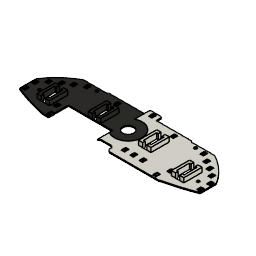
Amaturenbrett_Auto (Autodesk Fusion 360 design; units mm, degrees)
Autodesk Fusion 360 part; units mm, degrees
sketch "Skizze1" plane through (0, 0, 0) normal (0, 0, 1) x (1, 0, 0)
  line L0 (0, 10) -> (-10, 10)
  line L1 (-10, 10) -> (-13, 7)
  line L2 (-13, 7) -> (-13, 2)
  line L3 (-13, 2) -> (-15, 0)
  spline S0 degree 5 poles (-110, 0) (-110.1613, 0.0605) (-110.7348, 0.2373) (-112.3477, 0.67) (-115.9134, 1.5732) (-122.2237, 3.1932) (-129.7281, 5.2238) (-137.7121, 7.5525) (-145.4822, 10.0264) (-152.4484, 12.4304) (-158.1215, 14.5178) (-161.3098, 15.7444) (-162.8158, 16.3309) (-163.4105, 16.5624) (-163.6056, 16.6383) knots 0 0 0 0 0 0 0.1 0.2 0.3 0.4 0.5 0.6 0.7 0.8 0.9 1 1 1 1 1 1
  line L4 (-163.6056, 16.6383) -> (-163.6056, 46)
  spline S1 degree 5 poles (-163.6056, 46) (-163.4847, 46.1973) (-163.1089, 46.8) (-162.1433, 48.3283) (-160.053, 51.5223) (-156.1277, 56.9302) (-150.9771, 63.1091) (-144.7998, 69.3982) (-137.996, 75.2415) (-131.2216, 80.2701) (-125.2328, 84.2311) (-121.6617, 86.4119) (-119.9315, 87.445) (-119.2344, 87.8605) (-119, 88) knots 0 0 0 0 0 0 0.1 0.2 0.3 0.4 0.5 0.6 0.7 0.8 0.9 1 1 1 1 1 1
  line L5 (-119, 88) -> (-77, 88)
  line L6 (-77, 88) -> (-75, 90)
  line L7 (-75, 90) -> (-11, 90)
  line L8 (-11, 90) -> (-11, 99)
  line L9 (-11, 99) -> (-9.3607, 100.6393)
  line L10 (-9.3607, 100.6393) -> (0, 100.6393)
  line L11 (0, 1.75) -> (0, 22.5)
  line L12 (13, 2) -> (16.5, -1.5)
  line L13 (75, 90) -> (11, 90)
  line L14 (119, 88) -> (77, 88)
  spline S2 degree 5 poles (104.5, -1.5) (104.7668, -1.4344) (105.5646, -1.2376) (107.5534, -0.7459) (111.692, 0.289) (118.7937, 2.1326) (127.1068, 4.4102) (135.8553, 6.9754) (144.2868, 9.6506) (151.7717, 12.2139) (157.8159, 14.417) (161.1893, 15.7031) (162.777, 16.3168) (163.4017, 16.559) (163.6056, 16.6383) knots 0 0 0 0 0 0 0.1 0.2 0.3 0.4 0.5 0.6 0.7 0.8 0.9 1 1 1 1 1 1
  line L15 (-106, -1.5) -> (-114, 1.5)
  line L16 (-158.3876, 14.6077) -> (-168.8236, 18.669)
  line L17 (98.7017, -2.9261) -> (110.2983, -0.0739)
  line L18 (158.3876, 14.6077) -> (168.8236, 18.669)
  spline S3 degree 5 poles (163.6056, 46) (163.4847, 46.1973) (163.1089, 46.8) (162.1433, 48.3283) (160.053, 51.5223) (156.1277, 56.9302) (150.9771, 63.1091) (144.7998, 69.3982) (137.996, 75.2415) (131.2216, 80.2701) (125.2328, 84.2311) (121.6617, 86.4119) (119.9315, 87.445) (119.2344, 87.8605) (119, 88) knots 0 0 0 0 0 0 0.1 0.2 0.3 0.4 0.5 0.6 0.7 0.8 0.9 1 1 1 1 1 1
  line L19 (-167.0116, 40.4408) -> (-160.1996, 51.5592)
  line L20 (-125.039, 84.4076) -> (-112.961, 91.5924)
  line L21 (167.0116, 40.4408) -> (160.1996, 51.5592)
  line L22 (125.039, 84.4076) -> (112.961, 91.5924)
  line L23 (77, 88) -> (75, 90)
  line L24 (10, 10) -> (13, 7)
  line L25 (163.6056, 16.6383) -> (163.6056, 46)
  line L26 (16.5, -1.5) -> (104.5, -1.5)
  line L27 (11, 99) -> (9.3607, 100.6393)
  line L28 (13, 7) -> (13, 2)
  line L29 (0, 10) -> (10, 10)
  line L30 (9.3607, 100.6393) -> (0, 100.6393)
  line L31 (11, 90) -> (11, 99)
  circle A0 centre (-158.8575, 41.2647) radius 1.75
  circle A1 centre (-158.8575, 23.2647) radius 1.75
  circle A2 centre (-147.7393, 54.3878) radius 1.75
  circle A3 centre (-120.4151, 72.4981) radius 1.75
  circle A4 centre (158.8575, 23.2647) radius 1.75
  circle A5 centre (158.8575, 41.2647) radius 1.75
  circle A6 centre (0, 50) radius 25
  line L32 (11, 90) -> (11, 72.4499)
  line L33 (13, 7) -> (13, 28.6458)
  circle A7 centre (0, 50) radius 10
  circle A8 centre (-89.5, 82.5) radius 2.75
  circle A9 centre (143.3281, 32.327) radius 2.5
  circle A10 centre (-144.409, 32.4498) radius 2.5
  line L34 (-146.8803, 32.0722) -> (-144.8803, 32.0722)
  line L35 (-142.4192, 30.1189) -> (-142.2776, 30.1189)
  circle A11 centre (-106, 82) radius 1.75
  circle A12 centre (-103, 25) radius 1.75
  circle A13 centre (-95.8089, 4.2466) radius 1.75
  circle A14 centre (-45, 46) radius 5
  circle A15 centre (120.3035, 27.3959) radius 5
  line L36 (21.162, 34.5574) -> (76.9201, 34.5574)
  line L37 (76.9201, 34.5574) -> (76.9201, 2.4702)
  line L38 (76.9201, 2.4702) -> (21.162, 2.4702)
  line L39 (21.162, 2.4702) -> (21.162, 34.5574)
  line L40 (-110, 0) -> (-106, -1.5)
  line L41 (-106, -1.5) -> (-17, -1.5)
  line L42 (-17, -1.5) -> (-15, 0)
  circle A16 centre (-134.5283, 64.1132) radius 1.75
  line L43 (-161.8015, 26.3684) -> (-155.8015, 26.3684)
  line L44 (-155.8015, 26.3684) -> (-155.8015, 20.3684)
  line L45 (-155.8015, 20.3684) -> (-161.8015, 20.3684)
  line L46 (-161.8015, 20.3684) -> (-161.8015, 26.3684)
  line L47 (-161.7377, 38.3687) -> (-161.7377, 44.3687)
  line L48 (-161.7377, 44.3687) -> (-155.7377, 44.3687)
  line L49 (-155.7377, 44.3687) -> (-155.7377, 38.3687)
  line L50 (-155.7377, 38.3687) -> (-161.7377, 38.3687)
  line L51 (-131.5751, 61.1788) -> (-137.5751, 61.1788)
  line L52 (-137.5751, 61.1788) -> (-137.5751, 67.1788)
  line L53 (-137.5751, 67.1788) -> (-131.5751, 67.1788)
  line L54 (-131.5751, 67.1788) -> (-131.5751, 61.1788)
  line L55 (-123.3948, 69.6725) -> (-123.3948, 75.6725)
  line L56 (-123.3948, 75.6725) -> (-117.3948, 75.6725)
  line L57 (-117.3948, 75.6725) -> (-117.3948, 69.6725)
  line L58 (-117.3948, 69.6725) -> (-123.3948, 69.6725)
  line L59 (-108.9492, 79.0086) -> (-108.9492, 85.0086)
  line L60 (-108.9492, 85.0086) -> (-102.9492, 85.0086)
  line L61 (-102.9492, 85.0086) -> (-102.9492, 79.0086)
  line L62 (-102.9492, 79.0086) -> (-108.9492, 79.0086)
  line L63 (-106.0964, 22.0509) -> (-106.0964, 28.0509)
  line L64 (-106.0964, 28.0509) -> (-100.0964, 28.0509)
  line L65 (-100.0964, 28.0509) -> (-100.0964, 22.0509)
  line L66 (-100.0964, 22.0509) -> (-106.0964, 22.0509)
  line L67 (-98.7463, 7.3835) -> (-92.7463, 7.3835)
  line L68 (-92.7463, 7.3835) -> (-92.7463, 1.3835)
  line L69 (-92.7463, 1.3835) -> (-98.7463, 1.3835)
  line L70 (-98.7463, 1.3835) -> (-98.7463, 7.3835)
  circle A17 centre (-61.0017, 16.9954) radius 1.75
  line L71 (-63.9392, 13.9164) -> (-63.9392, 19.9164)
  line L72 (-57.9392, 13.9164) -> (-63.9392, 13.9164)
  line L73 (-57.9392, 19.9164) -> (-57.9392, 13.9164)
  line L74 (-63.9392, 19.9164) -> (-57.9392, 19.9164)
  circle A18 centre (-44.4166, 16.9103) radius 1.75
  circle A19 centre (-28.1708, 16.8342) radius 1.75
  line L75 (3.0172, 92.0677) -> (-2.9828, 92.0677)
  line L76 (-2.9828, 92.0677) -> (-2.9828, 98.0677)
  line L77 (-2.9828, 98.0677) -> (3.0172, 98.0677)
  line L78 (3.0172, 98.0677) -> (3.0172, 92.0677)
  circle A20 centre (0.0266, 95.0028) radius 1.75
  line L79 (-48.3744, 79.3302) -> (-54.3744, 79.3302)
  line L80 (-54.3744, 79.3302) -> (-54.3744, 85.3302)
  line L81 (-54.3744, 85.3302) -> (-48.3744, 85.3302)
  line L82 (-48.3744, 85.3302) -> (-48.3744, 79.3302)
  circle A21 centre (-51.3653, 82.3011) radius 1.75
  line L83 (47.6167, 79.2941) -> (47.6167, 85.2941)
  line L84 (47.6167, 85.2941) -> (53.6167, 85.2941)
  line L85 (53.6167, 85.2941) -> (53.6167, 79.2941)
  line L86 (53.6167, 79.2941) -> (47.6167, 79.2941)
  circle A22 centre (50.6982, 82.3011) radius 1.75
  circle A23 centre (89.1589, 82.4646) radius 2.5
  line L87 (102.0349, 78.6834) -> (102.0349, 84.6834)
  line L88 (102.0349, 84.6834) -> (108.0349, 84.6834)
  line L89 (108.0349, 84.6834) -> (108.0349, 78.6834)
  line L90 (108.0349, 78.6834) -> (102.0349, 78.6834)
  circle A24 centre (105.0444, 81.6905) radius 1.75
  line L91 (117.3503, 69.6133) -> (117.3503, 75.6133)
  line L92 (117.3503, 75.6133) -> (123.3503, 75.6133)
  line L93 (123.3503, 75.6133) -> (123.3503, 69.6133)
  line L94 (123.3503, 69.6133) -> (117.3503, 69.6133)
  circle A25 centre (120.4318, 72.5126) radius 1.75
  line L95 (130.8921, 61.2538) -> (130.8921, 67.2538)
  line L96 (130.8921, 67.2538) -> (136.8921, 67.2538)
  line L97 (136.8921, 67.2538) -> (136.8921, 61.2538)
  line L98 (136.8921, 61.2538) -> (130.8921, 61.2538)
  circle A26 centre (133.8942, 64.189) radius 1.75
  line L99 (150.7504, 51.4949) -> (144.7504, 51.4949)
  line L100 (144.7504, 51.4949) -> (144.7504, 57.4949)
  line L101 (144.7504, 57.4949) -> (150.7504, 57.4949)
  line L102 (150.7504, 57.4949) -> (150.7504, 51.4949)
  circle A27 centre (147.7239, 54.3795) radius 1.75
  line L103 (161.805, 38.5537) -> (155.805, 38.5537)
  line L104 (155.805, 38.5537) -> (155.805, 44.5537)
  line L105 (155.805, 44.5537) -> (161.805, 44.5537)
  line L106 (161.805, 44.5537) -> (161.805, 38.5537)
  line L107 (155.874, 26.4991) -> (161.874, 26.4991)
  line L108 (161.874, 26.4991) -> (161.874, 20.4991)
  line L109 (155.874, 20.4991) -> (155.874, 26.4991)
  line L110 (161.874, 20.4991) -> (155.874, 20.4991)
  circle A28 centre (95.7662, 4.2772) radius 1.75
  line L111 (92.7927, 7.3926) -> (98.7927, 7.3926)
  line L112 (98.7927, 7.3926) -> (98.7927, 1.3926)
  line L113 (92.7927, 1.3926) -> (92.7927, 7.3926)
  line L114 (98.7927, 1.3926) -> (92.7927, 1.3926)
  line L115 (106.0344, 22.2433) -> (100.0344, 22.2433)
  line L116 (100.0344, 22.2433) -> (100.0344, 28.2433)
  line L117 (100.0344, 28.2433) -> (106.0344, 28.2433)
  line L118 (106.0344, 28.2433) -> (106.0344, 22.2433)
  circle A29 centre (103.0079, 25.128) radius 1.75
  line L119 (-144.7191, 51.5389) -> (-150.7191, 51.5389)
  line L120 (-150.7191, 51.5389) -> (-150.7191, 57.5389)
  line L121 (-150.7191, 57.5389) -> (-144.7191, 57.5389)
  line L122 (-144.7191, 57.5389) -> (-144.7191, 51.5389)
  line L123 (-41.4351, 13.9164) -> (-47.4351, 13.9164)
  line L124 (-47.4351, 13.9164) -> (-47.4351, 19.9164)
  line L125 (-47.4351, 19.9164) -> (-41.4351, 19.9164)
  line L126 (-41.4351, 19.9164) -> (-41.4351, 13.9164)
  line L127 (-25.4351, 13.9164) -> (-31.4351, 13.9164)
  line L128 (-31.4351, 13.9164) -> (-31.4351, 19.9164)
  line L129 (-31.4351, 19.9164) -> (-25.4351, 19.9164)
  line L130 (-25.4351, 19.9164) -> (-25.4351, 13.9164)
  line L131 (-38.3249, 39.7163) -> (-51.8249, 39.7163)
  line L132 (-51.8249, 39.7163) -> (-51.8249, 63.2163)
  line L133 (-51.8249, 63.2163) -> (-38.3249, 63.2163)
  line L134 (-38.3249, 63.2163) -> (-38.3249, 39.7163)
  line L135 (-38.3249, 39.9465) -> (-38.3249, 63.2163)
  line L136 (-56.2684, 39.9376) -> (-56.2684, 62.9381)
  line L137 (-33.7684, 67.9381) -> (-56.2684, 67.9381)
  line L138 (-56.2684, 67.9381) -> (-56.2684, 62.9381)
  line L139 (-33.7684, 34.9376) -> (-56.2684, 34.9376)
  line L140 (-56.2684, 34.9376) -> (-56.2684, 39.9376)
  line L141 (-33.7684, 67.9381) -> (-56.2684, 67.9381)
  line L142 (-56.2684, 67.9381) -> (-56.2684, 62.9381)
  line L143 (-56.2684, 34.9376) -> (-56.2684, 39.9376)
  line L144 (-33.7684, 34.9376) -> (-56.2684, 34.9376)
  line L145 (-33.7684, 34.9376) -> (-33.7684, 67.9381)
  line L146 (39.1751, 39.7163) -> (39.1751, 63.2163)
  line L147 (39.1751, 63.2163) -> (52.6751, 63.2163)
  line L148 (34.7316, 34.9376) -> (34.7316, 39.9376)
  line L149 (57.2316, 34.9376) -> (34.7316, 34.9376)
  line L150 (52.6751, 63.2163) -> (52.6751, 39.7163)
  line L151 (57.2316, 67.9381) -> (34.7316, 67.9381)
  line L152 (57.2316, 34.9376) -> (57.2316, 67.9381)
  line L153 (52.6751, 39.7163) -> (39.1751, 39.7163)
  circle A30 centre (46, 46) radius 5
  line L154 (34.7316, 39.9376) -> (34.7316, 62.9381)
  line L155 (34.7316, 67.9381) -> (34.7316, 62.9381)
  line L156 (57.2316, 67.9381) -> (34.7316, 67.9381)
  line L157 (57.2316, 34.9376) -> (34.7316, 34.9376)
  line L158 (34.7316, 34.9376) -> (34.7316, 39.9376)
  line L159 (52.6751, 39.9465) -> (52.6751, 63.2163)
  line L160 (34.7316, 67.9381) -> (34.7316, 62.9381)
  line L161 (-33.7684, 34.9376) -> (-33.7684, 67.9381)
  line L162 (-33.7684, 34.9376) -> (-56.2684, 34.9376)
  line L163 (-56.2684, 34.9376) -> (-56.2684, 39.9376)
  line L164 (-56.2684, 39.9376) -> (-56.2684, 62.9381)
  line L165 (-56.2684, 67.9381) -> (-56.2684, 62.9381)
  line L166 (-33.7684, 67.9381) -> (-56.2684, 67.9381)
  line L167 (-38.3249, 63.2163) -> (-38.3249, 39.7163)
  line L168 (-51.8249, 39.7163) -> (-51.8249, 63.2163)
  line L169 (-51.8249, 63.2163) -> (-38.3249, 63.2163)
  line L170 (-38.3249, 39.7163) -> (-51.8249, 39.7163)
  line L171 (-33.7684, 34.9376) -> (-33.7684, 67.9381)
  line L172 (-33.7684, 34.9376) -> (-56.2684, 34.9376)
  line L173 (-56.2684, 34.9376) -> (-56.2684, 39.9376)
  line L174 (-56.2684, 39.9376) -> (-56.2684, 62.9381)
  line L175 (-56.2684, 67.9381) -> (-56.2684, 62.9381)
  line L176 (-33.7684, 67.9381) -> (-56.2684, 67.9381)
  line L177 (-51.8249, 63.2163) -> (-38.3249, 63.2163)
  line L178 (-38.3249, 63.2163) -> (-38.3249, 39.7163)
  line L179 (-51.8249, 39.7163) -> (-51.8249, 63.2163)
  line L180 (-38.3249, 39.7163) -> (-51.8249, 39.7163)
  circle A31 centre (-122.3546, 28.1544) radius 5
  line L181 (-133.6684, 17.0376) -> (-133.6684, 22.0376)
  line L182 (-133.6684, 20.0376) -> (-133.6684, 45.0381)
  line L183 (-133.6684, 50.0381) -> (-133.6684, 45.0381)
  line L184 (-111.1684, 50.0381) -> (-133.6684, 50.0381)
  line L185 (-111.1684, 17.0376) -> (-111.1684, 50.0381)
  line L186 (-111.1684, 17.0376) -> (-133.6684, 17.0376)
  line L187 (-133.6684, 15.0376) -> (-133.6684, 20.0376)
  line L188 (-129.2249, 45.3163) -> (-115.7249, 45.3163)
  line L189 (-115.7249, 45.3163) -> (-115.7249, 21.8163)
  line L190 (-129.2249, 21.8163) -> (-129.2249, 45.3163)
  line L191 (-115.7249, 21.8163) -> (-129.2249, 21.8163)
  line L192 (109.0526, 21.3481) -> (109.0526, 44.3486)
  line L193 (109.0526, 16.3481) -> (109.0526, 21.3481)
  line L194 (131.5526, 16.3481) -> (109.0526, 16.3481)
  line L195 (131.5526, 16.3481) -> (131.5526, 49.3486)
  line L196 (131.5526, 49.3486) -> (109.0526, 49.3486)
  line L197 (109.0526, 49.3486) -> (109.0526, 44.3486)
  line L198 (126.9961, 21.1268) -> (113.4961, 21.1268)
  line L199 (113.4961, 21.1268) -> (113.4961, 44.6268)
  line L200 (113.4961, 44.6268) -> (126.9961, 44.6268)
  line L201 (126.9961, 44.6268) -> (126.9961, 21.1268)
  line L202 (116.5254, 44.6268) -> (116.5254, 49.3486)
  line L203 (123.9565, 44.6268) -> (123.9565, 49.3486)
  line L204 (116.5254, 44.6268) -> (116.5254, 16.3481)
  line L205 (123.9565, 49.3486) -> (123.9565, 16.3481)
  line L206 (120.2461, 44.6268) -> (116.5461, 44.6268)
  line L207 (123.9565, 44.6268) -> (123.9565, 49.3486)
  line L208 (123.9565, 49.3486) -> (123.9565, 16.3481)
  line L209 (116.5254, 44.6268) -> (116.5254, 49.3486)
  line L210 (116.5254, 44.6268) -> (116.5254, 16.3481)
  line L211 (45.9251, 63.2163) -> (49.6251, 63.2163)
  line L212 (45.9251, 63.2163) -> (42.2251, 63.2163)
  line L213 (42.2251, 63.2163) -> (42.2251, 67.9381)
  line L214 (42.2251, 67.9381) -> (42.2251, 34.9376)
  line L215 (49.6251, 67.9381) -> (49.6251, 34.9376)
  line L216 (-45.0184, 67.9381) -> (-48.7184, 67.9381)
  line L217 (-45.0184, 67.9381) -> (-41.3184, 67.9381)
  line L218 (-41.3184, 67.9381) -> (-41.3184, 34.9376)
  line L219 (-48.7184, 67.9381) -> (-48.7184, 34.9376)
  line L220 (-122.4184, 50.0381) -> (-126.1184, 50.0381)
  line L221 (-122.4184, 50.0381) -> (-118.7184, 50.0381)
  line L222 (-126.1184, 50.0381) -> (-126.1184, 17.0376)
  line L223 (-118.7184, 50.0381) -> (-118.7184, 17.0376)
  line L224 (13, -1.5) -> (92.9118, -1.5)
  line L225 (92.9118, -1.5) -> (92.9118, 34.5574)
  line L226 (92.9118, 34.5574) -> (13, 34.5574)
  line L227 (13, 34.5574) -> (13, -1.5)
  line L228 (-54.3744, 79.3302) -> (-48.3744, 79.3302)
  line L229 (-48.3744, 79.3302) -> (-48.3744, 77.3302)
  line L230 (-48.3744, 77.3302) -> (-54.3744, 77.3302)
  line L231 (-54.3744, 77.3302) -> (-54.3744, 79.3302)
  line L232 (-102.9492, 79.0086) -> (-108.9492, 79.0086)
  line L233 (-108.9492, 79.0086) -> (-108.9492, 77.0086)
  line L234 (-108.9492, 77.0086) -> (-102.9492, 77.0086)
  line L235 (-102.9492, 77.0086) -> (-102.9492, 79.0086)
  line L236 (-117.3948, 69.6725) -> (-123.3948, 69.6725)
  line L237 (-123.3948, 69.6725) -> (-123.3948, 67.6725)
  line L238 (-123.3948, 67.6725) -> (-117.3948, 67.6725)
  line L239 (-117.3948, 67.6725) -> (-117.3948, 69.6725)
  line L240 (-131.5751, 61.1788) -> (-137.5751, 61.1788)
  line L241 (-137.5751, 61.1788) -> (-137.5751, 59.1788)
  line L242 (-137.5751, 59.1788) -> (-131.5751, 59.1788)
  line L243 (-131.5751, 59.1788) -> (-131.5751, 61.1788)
  line L244 (-144.7191, 51.5389) -> (-150.7191, 51.5389)
  line L245 (-150.7191, 51.5389) -> (-150.7191, 49.5389)
  line L246 (-150.7191, 49.5389) -> (-144.7191, 49.5389)
  line L247 (-144.7191, 49.5389) -> (-144.7191, 51.5389)
  line L248 (-155.7377, 38.3687) -> (-161.7377, 38.3687)
  line L249 (-161.7377, 38.3687) -> (-161.7377, 36.3687)
  line L250 (-161.7377, 36.3687) -> (-155.7377, 36.3687)
  line L251 (-155.7377, 36.3687) -> (-155.7377, 38.3687)
  line L252 (-155.8015, 20.3684) -> (-161.8015, 20.3684)
  line L253 (-161.8015, 20.3684) -> (-161.8015, 18.3684)
  line L254 (-161.8015, 18.3684) -> (-155.8015, 18.3684)
  line L255 (-155.8015, 18.3684) -> (-155.8015, 20.3684)
  line L256 (-100.0964, 22.0509) -> (-106.0964, 22.0509)
  line L257 (-106.0964, 22.0509) -> (-106.0964, 20.0509)
  line L258 (-106.0964, 20.0509) -> (-100.0964, 20.0509)
  line L259 (-100.0964, 20.0509) -> (-100.0964, 22.0509)
  line L260 (-92.7463, 7.3835) -> (-98.7463, 7.3835)
  line L261 (-98.7463, 7.3835) -> (-98.7463, 9.3835)
  line L262 (-98.7463, 9.3835) -> (-92.7463, 9.3835)
  line L263 (-92.7463, 9.3835) -> (-92.7463, 7.3835)
  line L264 (-63.9392, 13.9164) -> (-57.9392, 13.9164)
  line L265 (-57.9392, 13.9164) -> (-57.9392, 11.9164)
  line L266 (-57.9392, 11.9164) -> (-63.9392, 11.9164)
  line L267 (-63.9392, 11.9164) -> (-63.9392, 13.9164)
  line L268 (-47.4351, 13.9164) -> (-41.4351, 13.9164)
  line L269 (-41.4351, 13.9164) -> (-41.4351, 11.9164)
  line L270 (-41.4351, 11.9164) -> (-47.4351, 11.9164)
  line L271 (-47.4351, 11.9164) -> (-47.4351, 13.9164)
  line L272 (-31.4351, 13.9164) -> (-25.4351, 13.9164)
  line L273 (-25.4351, 13.9164) -> (-25.4351, 11.9164)
  line L274 (-25.4351, 11.9164) -> (-31.4351, 11.9164)
  line L275 (-31.4351, 11.9164) -> (-31.4351, 13.9164)
  line L276 (47.6167, 79.2941) -> (53.6167, 79.2941)
  line L277 (53.6167, 79.2941) -> (53.6167, 77.2941)
  line L278 (53.6167, 77.2941) -> (47.6167, 77.2941)
  line L279 (47.6167, 77.2941) -> (47.6167, 79.2941)
  line L280 (102.0349, 78.6834) -> (108.0349, 78.6834)
  line L281 (108.0349, 78.6834) -> (108.0349, 76.6834)
  line L282 (108.0349, 76.6834) -> (102.0349, 76.6834)
  line L283 (102.0349, 76.6834) -> (102.0349, 78.6834)
  line L284 (117.3503, 69.6133) -> (123.3503, 69.6133)
  line L285 (123.3503, 69.6133) -> (123.3503, 67.6133)
  line L286 (123.3503, 67.6133) -> (117.3503, 67.6133)
  line L287 (117.3503, 67.6133) -> (117.3503, 69.6133)
  line L288 (130.8921, 61.2538) -> (136.8921, 61.2538)
  line L289 (136.8921, 61.2538) -> (136.8921, 59.2538)
  line L290 (136.8921, 59.2538) -> (130.8921, 59.2538)
  line L291 (130.8921, 59.2538) -> (130.8921, 61.2538)
  line L292 (144.7504, 51.4949) -> (150.7504, 51.4949)
  line L293 (150.7504, 51.4949) -> (150.7504, 49.4949)
  line L294 (150.7504, 49.4949) -> (144.7504, 49.4949)
  line L295 (144.7504, 49.4949) -> (144.7504, 51.4949)
  line L296 (155.805, 38.5537) -> (161.805, 38.5537)
  line L297 (161.805, 38.5537) -> (161.805, 36.5537)
  line L298 (161.805, 36.5537) -> (155.805, 36.5537)
  line L299 (155.805, 36.5537) -> (155.805, 38.5537)
  line L300 (155.874, 20.4991) -> (161.874, 20.4991)
  line L301 (161.874, 20.4991) -> (161.874, 18.4991)
  line L302 (161.874, 18.4991) -> (155.874, 18.4991)
  line L303 (155.874, 18.4991) -> (155.874, 20.4991)
  line L304 (100.0344, 22.2433) -> (106.0344, 22.2433)
  line L305 (106.0344, 22.2433) -> (106.0344, 20.2433)
  line L306 (106.0344, 20.2433) -> (100.0344, 20.2433)
  line L307 (100.0344, 20.2433) -> (100.0344, 22.2433)
  line L308 (98.7927, 7.3926) -> (92.7927, 7.3926)
  line L309 (92.7927, 7.3926) -> (92.7927, 9.3926)
  line L310 (92.7927, 9.3926) -> (98.7927, 9.3926)
  line L311 (98.7927, 9.3926) -> (98.7927, 7.3926)
  line L312 (3.0172, 92.0677) -> (-2.9828, 92.0677)
  line L313 (-2.9828, 92.0677) -> (-2.9828, 90.0677)
  line L314 (-2.9828, 90.0677) -> (3.0172, 90.0677)
  line L315 (3.0172, 90.0677) -> (3.0172, 92.0677)
  point P0 (-139, 8)
  point P1 (-146, 68)
  point P2 (146, 68)
  point P3 (139, 8)
  point P4 (-120.6376, 72.9849)
  point P5 (-85, 76)
  point P6 (-120.6376, 72.9849)
  dimension "d3" = 3.5
  dimension "d4" = 3.5
  dimension "d5" = 3.5
  dimension "d6" = 3.5
  dimension "d15" = 20
  dimension "d23" = 5.5
  dimension "d35" = 5
  dimension "d37" = 2
  dimension "d38" = 5
  dimension "d39" = 3.5
  dimension "d41" = 3.5
  dimension "d46" = 3.5
  dimension "d52" = 10
  dimension "d54" = 10
  dimension "d55" = 3.5
  dimension "d60" = 6
  dimension "d61" = 6
  dimension "d62" = 6
  dimension "d63" = 6
  dimension "d66" = 6
  dimension "d67" = 6
  dimension "d68" = 6
  dimension "d69" = 6
  dimension "d70" = 6
  dimension "d71" = 6
  dimension "d72" = 6
  dimension "d73" = 6
  dimension "d74" = 6
  dimension "d75" = 6
  dimension "d76" = 3.5
  dimension "d77" = 6
  dimension "d78" = 6
  dimension "d79" = 3.5
  dimension "d82" = 3.5
  dimension "d85" = 3.5
  dimension "d86" = 6
  dimension "d87" = 6
  dimension "d88" = 3.5
  dimension "d89" = 6
  dimension "d90" = 6
  dimension "d91" = 3.5
  dimension "d92" = 6
  dimension "d93" = 6
  dimension "d94" = 5
  dimension "d97" = 3.5
  dimension "d98" = 6
  dimension "d99" = 6
  dimension "d100" = 3.5
  dimension "d101" = 6
  dimension "d102" = 6
  dimension "d103" = 3.5
  dimension "d104" = 6
  dimension "d105" = 6
  dimension "d106" = 3.5
  dimension "d107" = 6
  dimension "d108" = 6
  dimension "d109" = 6
  dimension "d110" = 6
  dimension "d111" = 6
  dimension "d112" = 6
  dimension "d113" = 3.5
  dimension "d114" = 6
  dimension "d115" = 6
  dimension "d116" = 3.5
  dimension "d117" = 6
  dimension "d118" = 6
  dimension "d137" = 6
  dimension "d138" = 6
  dimension "d139" = 6
  dimension "d140" = 6
  dimension "d141" = 6
  dimension "d142" = 6
  dimension "d149" = 13.5
  dimension "d150" = 23.5
  dimension "d160" = 5
  dimension "d162" = 5
  dimension "d164" = 5
  dimension "d166" = 5
  dimension "d171" = 10
  dimension "d172" = 13.5
  dimension "d173" = 23.5
  dimension "d174" = 5
  dimension "d175" = 5
  dimension "d176" = 5
  dimension "d177" = 5
  dimension "d180" = 13.5
  dimension "d181" = 23.5
  dimension "d182" = 5
  dimension "d183" = 5
  dimension "d184" = 10
  dimension "d185" = 13.5
  dimension "d186" = 23.5
  dimension "d187" = 5
  dimension "d188" = 5
  dimension "d190" = 5
  dimension "d191" = 5
  dimension "d192" = 5
  dimension "d193" = 13.5
  dimension "d194" = 23.5
  dimension "d196" = 13.5
  dimension "d197" = 23.5
  dimension "d198" = 5
  dimension "d199" = 5
  dimension "d200" = 3.7
  dimension "d201" = 3.7
  dimension "d202" = 3.7
  dimension "d203" = 3.7
  dimension "d204" = 3.7
  dimension "d205" = 3.7
  dimension "d206" = 3.7
  dimension "d207" = 2
  dimension "d208" = 2
  dimension "d209" = 2
  dimension "d210" = 6
  dimension "d211" = 2
  dimension "d212" = 2
  dimension "d213" = 2
  dimension "d214" = 2
  dimension "d215" = 2
  dimension "d216" = 6
  dimension "d217" = 2
  dimension "d218" = 2
  dimension "d219" = 2
  dimension "d220" = 2
  dimension "d221" = 6
  dimension "d222" = 2
  dimension "d223" = 6
  dimension "d224" = 2
  dimension "d225" = 2
  dimension "d226" = 2
  dimension "d227" = 6
  dimension "d228" = 2
  dimension "d229" = 2
  dimension "d230" = 2
  dimension "d231" = 2
  dimension "d232" = 6
  dimension "d233" = 2
  dimension "d234" = 2
  constraint horizontal L0
  constraint vertical L2
  constraint parallel L1 L3
  constraint vertical L4
  constraint horizontal L5
  constraint parallel L5 L7
  constraint perpendicular L7 L8
  constraint parallel L6 L9
  constraint parallel L7 L10
  constraint midpoint S0.start L15
  constraint midpoint S0.end L16
  constraint midpoint L4.end L19
  constraint midpoint S1.end L20
  constraint symmetric L11 A0 A5
  constraint symmetric L11 A1 A4
  constraint coincident A6 L32.end
  constraint perpendicular L13 L32
  constraint coincident A6 L33.end
  constraint parallel L28 L33
  constraint concentric A6 A7
  constraint horizontal L34
  constraint horizontal L35
  constraint coincident L34.start A10
  constraint vertical L37
  constraint horizontal L38
  constraint vertical L39
  constraint coincident L15.start L40.end
  constraint parallel L15 L40
  constraint midpoint S2.start L17
  constraint horizontal L43
  constraint vertical L44
  constraint horizontal L45
  constraint vertical L46
  constraint horizontal L48
  constraint vertical L49
  constraint horizontal L50
  constraint vertical L47
  constraint horizontal L53
  constraint vertical L54
  constraint horizontal L51
  constraint vertical L52
  constraint horizontal L56
  constraint vertical L57
  constraint horizontal L58
  constraint vertical L55
  constraint horizontal L60
  constraint vertical L61
  constraint horizontal L62
  constraint vertical L59
  constraint horizontal L64
  constraint vertical L65
  constraint horizontal L66
  constraint vertical L63
  constraint horizontal L67
  constraint vertical L68
  constraint horizontal L69
  constraint vertical L70
  constraint horizontal L74
  constraint vertical L73
  constraint horizontal L72
  constraint vertical L71
  constraint horizontal L77
  constraint vertical L78
  constraint horizontal L75
  constraint vertical L76
  constraint horizontal L81
  constraint vertical L82
  constraint horizontal L79
  constraint vertical L80
  constraint horizontal L84
  constraint vertical L85
  constraint horizontal L86
  constraint vertical L83
  constraint horizontal L88
  constraint vertical L89
  constraint horizontal L90
  constraint vertical L87
  constraint horizontal L92
  constraint vertical L93
  constraint horizontal L94
  constraint vertical L91
  constraint horizontal L96
  constraint vertical L97
  constraint horizontal L98
  constraint vertical L95
  constraint horizontal L101
  constraint vertical L102
  constraint horizontal L99
  constraint vertical L100
  constraint horizontal L105
  constraint vertical L106
  constraint horizontal L103
  constraint vertical L104
  constraint horizontal L107
  constraint vertical L108
  constraint horizontal L110
  constraint vertical L109
  constraint horizontal L111
  constraint vertical L112
  constraint horizontal L114
  constraint vertical L113
  constraint horizontal L117
  constraint vertical L118
  constraint horizontal L115
  constraint vertical L116
  constraint horizontal L121
  constraint vertical L122
  constraint horizontal L119
  constraint vertical L120
  constraint horizontal L125
  constraint vertical L126
  constraint horizontal L123
  constraint vertical L124
  constraint horizontal L129
  constraint vertical L130
  constraint horizontal L127
  constraint vertical L128
  constraint horizontal L133
  constraint vertical L134
  constraint horizontal L131
  constraint vertical L132
  constraint vertical L135
  constraint vertical L136
  constraint horizontal L137
  constraint vertical L138
  constraint horizontal L139
  constraint vertical L140
  constraint horizontal L141
  constraint vertical L142
  constraint horizontal L144
  constraint vertical L143
  constraint perpendicular L137 L145
  constraint horizontal L147
  constraint vertical L150
  constraint horizontal L153
  constraint vertical L146
  constraint vertical L159
  constraint vertical L154
  constraint horizontal L156
  constraint vertical L155
  constraint horizontal L149
  constraint vertical L158
  constraint horizontal L151
  constraint vertical L160
  constraint horizontal L157
  constraint vertical L148
  constraint perpendicular L152 L156
  constraint horizontal L169
  constraint vertical L167
  constraint horizontal L170
  constraint vertical L168
  constraint vertical L164
  constraint horizontal L166
  constraint vertical L165
  constraint horizontal L162
  constraint vertical L163
  constraint perpendicular L161 L166
  constraint horizontal L177
  constraint vertical L178
  constraint horizontal L180
  constraint vertical L179
  constraint vertical L174
  constraint horizontal L176
  constraint vertical L175
  constraint horizontal L172
  constraint vertical L173
  constraint perpendicular L171 L176
  constraint vertical L182
  constraint horizontal L184
  constraint vertical L183
  constraint vertical L187
  constraint horizontal L186
  constraint vertical L181
  constraint perpendicular L184 L185
  constraint horizontal L188
  constraint vertical L189
  constraint horizontal L191
  constraint vertical L190
  constraint horizontal L200
  constraint vertical L201
  constraint horizontal L198
  constraint vertical L199
  constraint vertical L192
  constraint horizontal L196
  constraint vertical L197
  constraint horizontal L194
  constraint vertical L193
  constraint perpendicular L195 L196
  constraint coincident L200 L202.start
  constraint coincident L196 L202.end
  constraint perpendicular L196 L202
  constraint coincident L200 L203.start
  constraint coincident L196 L203.end
  constraint perpendicular L196 L203
  constraint coincident L194 L204.end
  constraint perpendicular L194 L204
  constraint coincident L194 L205.end
  constraint perpendicular L194 L205
  constraint midpoint L200 L206.start
  constraint perpendicular L204 L206
  constraint midpoint L147 L211.start
  constraint parallel L147 L211
  constraint perpendicular L146 L212
  constraint coincident L156 L213.end
  constraint perpendicular L156 L213
  constraint coincident L149 L214.end
  constraint perpendicular L149 L214
  constraint coincident L156 L215.start
  constraint perpendicular L153 L215
  constraint midpoint L137 L216.start
  constraint perpendicular L142 L216
  constraint parallel L141 L217
  constraint coincident L139 L218.end
  constraint perpendicular L139 L218
  constraint coincident L172 L219.end
  constraint perpendicular L172 L219
  constraint midpoint L184 L220.start
  constraint parallel L184 L220
  constraint perpendicular L183 L221
  constraint coincident L186 L222.end
  constraint perpendicular L186 L222
  constraint coincident L186 L223.end
  constraint perpendicular L186 L223
  constraint horizontal L224
  constraint vertical L225
  constraint horizontal L226
  constraint vertical L227
  constraint horizontal L228
  constraint vertical L229
  constraint horizontal L230
  constraint vertical L231
  constraint horizontal L232
  constraint vertical L233
  constraint horizontal L234
  constraint vertical L235
  constraint horizontal L236
  constraint vertical L237
  constraint horizontal L238
  constraint vertical L239
  constraint horizontal L240
  constraint vertical L241
  constraint horizontal L242
  constraint vertical L243
  constraint horizontal L244
  constraint vertical L245
  constraint horizontal L246
  constraint vertical L247
  constraint horizontal L248
  constraint vertical L249
  constraint horizontal L250
  constraint vertical L251
  constraint horizontal L252
  constraint vertical L253
  constraint horizontal L254
  constraint vertical L255
  constraint horizontal L256
  constraint vertical L257
  constraint horizontal L258
  constraint vertical L259
  constraint horizontal L260
  constraint vertical L261
  constraint horizontal L262
  constraint vertical L263
  constraint horizontal L264
  constraint vertical L265
  constraint horizontal L266
  constraint vertical L267
  constraint horizontal L268
  constraint vertical L269
  constraint horizontal L270
  constraint vertical L271
  constraint horizontal L272
  constraint vertical L273
  constraint horizontal L274
  constraint vertical L275
  constraint horizontal L276
  constraint vertical L277
  constraint horizontal L278
  constraint vertical L279
  constraint horizontal L280
  constraint vertical L281
  constraint horizontal L282
  constraint vertical L283
  constraint horizontal L284
  constraint vertical L285
  constraint horizontal L286
  constraint vertical L287
  constraint horizontal L288
  constraint vertical L289
  constraint horizontal L290
  constraint vertical L291
  constraint horizontal L292
  constraint vertical L293
  constraint horizontal L294
  constraint vertical L295
  constraint horizontal L296
  constraint vertical L297
  constraint horizontal L298
  constraint vertical L299
  constraint horizontal L300
  constraint vertical L301
  constraint horizontal L302
  constraint vertical L303
  constraint horizontal L304
  constraint vertical L305
  constraint horizontal L306
  constraint vertical L307
  constraint horizontal L308
  constraint vertical L309
  constraint horizontal L310
  constraint vertical L311
  constraint horizontal L312
  constraint vertical L313
  constraint horizontal L314
  constraint vertical L315
  measures "d3" diameter of A0
  measures "d4" diameter of A1
  measures "d5" diameter of A2
  measures "d6" diameter of A3
  measures "d15" diameter of A7
  measures "d23" diameter of A8
  measures "d35" diameter of A10
  measures "d37" distance of L34.end L34.start
  measures "d38" distance of L35.end L34.start
  measures "d39" diameter of A11
  measures "d41" diameter of A12
  measures "d46" diameter of A13
  measures "d52" diameter of A14
  measures "d54" diameter of A15
  measures "d55" diameter of A16
  measures "d60" distance of L43.start L43.end
  measures "d61" distance of L43.start L45.end
  measures "d62" distance of L47.end L48.end
  measures "d63" distance of L47.end L47.start
  measures "d66" distance of L52.end L53.end
  measures "d67" distance of L52.end L51.end
  measures "d68" distance of L55.end L56.end
  measures "d69" distance of L55.end L55.start
  measures "d70" distance of L60.end L59.end
  measures "d71" distance of L59.start L59.end
  measures "d72" distance of L63.end L64.end
  measures "d73" distance of L63.end L63.start
  measures "d74" distance of L67.start L67.end
  measures "d75" distance of L67.start L69.end
  measures "d76" diameter of A17
  measures "d77" distance of L71.end L73.start
  measures "d78" distance of L71.end L71.start
  measures "d79" diameter of A18
  measures "d82" diameter of A19
  measures "d85" diameter of A20
  measures "d86" distance of L76.end L77.end
  measures "d87" distance of L76.end L75.end
  measures "d88" diameter of A21
  measures "d89" distance of L80.end L81.end
  measures "d90" distance of L79.end L80.end
  measures "d91" diameter of A22
  measures "d92" distance of L83.end L84.end
  measures "d93" distance of L83.end L83.start
  measures "d94" diameter of A23
  measures "d97" diameter of A24
  measures "d98" distance of L87.end L88.end
  measures "d99" distance of L87.end L87.start
  measures "d100" diameter of A25
  measures "d101" distance of L91.end L92.end
  measures "d102" distance of L91.start L91.end
  measures "d103" diameter of A26
  measures "d104" distance of L96.end L95.end
  measures "d105" distance of L95.start L95.end
  measures "d106" diameter of A27
  measures "d107" distance of L100.end L101.end
  measures "d108" distance of L100.end L99.end
  measures "d109" distance of L104.end L105.end
  measures "d110" distance of L104.end L103.end
  measures "d111" distance of L107.start L107.end
  measures "d112" distance of L109.start L107.start
  measures "d113" diameter of A28
  measures "d114" distance of L111.start L111.end
  measures "d115" distance of L111.start L113.start
  measures "d116" diameter of A29
  measures "d117" distance of L116.end L117.end
  measures "d118" distance of L116.end L115.end
  measures "d137" distance of L120.end L121.end
  measures "d138" distance of L120.end L119.end
  measures "d139" distance of L124.end L125.end
  measures "d140" distance of L124.end L123.end
  measures "d141" distance of L128.end L129.end
  measures "d142" distance of L128.end L127.end
  measures "d149" distance of L133.end L132.end
  measures "d150" distance of L131.end L132.end
  measures "d160" distance of L136.end L137.end
  measures "d162" distance of L136.start L139.end
  measures "d164" distance of L137.end L136.end
  measures "d166" distance of L139.end L136.start
  measures "d171" diameter of A30
  measures "d172" distance of L146.end L147.end
  measures "d173" distance of L146.end L146.start
  measures "d174" distance of L154.end L151.end
  measures "d175" distance of L148.end L148.start
  measures "d176" distance of L151.end L154.end
  measures "d177" distance of L148.start L148.end
  measures "d180" distance of L132.end L133.end
  measures "d181" distance of L131.end L132.end
  measures "d182" distance of L136.end L137.end
  measures "d183" distance of L139.end L136.start
  measures "d184" diameter of A31
  measures "d185" distance of L132.end L133.end
  measures "d186" distance of L131.end L132.end
  measures "d187" distance of L136.end L137.end
  measures "d188" distance of L139.end L136.start
  measures "d190" distance of L182.end L183.start
  measures "d191" distance of L187.start L182.start
  measures "d192" distance of L181.end L181.start
  measures "d193" distance of L188.start L188.end
  measures "d194" distance of L190.start L188.start
  measures "d196" distance of L199.end L200.end
  measures "d197" distance of L199.end L198.end
  measures "d198" distance of L192.end L196.end
  measures "d199" distance of L193.start L192.start
  measures "d200" distance of L206.start L206.end
  measures "d201" distance of L211.start L211.end
  measures "d202" distance of L211.start L212.end
  measures "d203" distance of L216.start L216.end
  measures "d204" distance of L216.start L217.end
  measures "d205" distance of L220.start L220.end
  measures "d206" distance of L220.start L221.end
  measures "d207" distance of L79.end L230.end
  measures "d208" distance of L61.end L234.end
  measures "d209" distance of L57.end L238.end
  measures "d210" distance of L51.start L51.end
  measures "d211" distance of L51.start L242.end
  measures "d212" distance of L119.start L246.end
  measures "d213" distance of L49.end L250.end
  measures "d214" distance of L44.end L254.end
  measures "d215" distance of L65.end L258.end
  measures "d216" distance of L67.end L67.start
  measures "d217" distance of L67.end L262.end
  measures "d218" distance of L71.start L266.end
  measures "d219" distance of L123.end L270.end
  measures "d220" distance of L127.end L274.end
  measures "d221" distance of L83.start L85.end
  measures "d222" distance of L83.start L278.end
  measures "d223" distance of L87.start L89.end
  measures "d224" distance of L87.start L282.end
  measures "d225" distance of L91.start L286.end
  measures "d226" distance of L95.start L290.end
  measures "d227" distance of L99.end L99.start
  measures "d228" distance of L99.end L294.end
  measures "d229" distance of L103.end L298.end
  measures "d230" distance of L109.start L302.end
  measures "d231" distance of L115.end L306.end
  measures "d232" distance of L111.end L111.start
  measures "d233" distance of L111.end L310.end
  measures "d234" distance of L75.start L314.end
extrude "Extrusion2" add sketch "Skizze1" along normal blind 2 contours A6 L226 L227 | L13 L14 S2 S3 L23 L25 L26 A6 L32 L36 L112 L114 L225 L226 L310 L311 | L111 L112 L114 L225 L308 | L111 L113 L114 L225 L308 | L111 L225 L308 L310 L311 | L194 L195 L196 L198 L200 L201 L203 L205 L207 L208 | L192 L193 L194 L196 L197 L198 L199 L200 L202 L204 L209 L210 | L83 L84 L85 L86 L276 | L86 L276 L277 L278 L279 | L87 L88 L89 L90 L280 | L90 L280 L281 L282 L283 | L91 L92 L93 L94 L284 | L94 L284 L285 L286 L287 | L95 L96 L97 L98 L288 | L98 L288 L289 L290 L291 | L99 L292 L293 L294 L295 | L99 L100 L101 L102 L292 | L103 L296 L297 L298 L299 | L103 L104 L105 L106 L296 | L107 L108 L109 L110 L300 | L110 L300 L301 L302 L303 | L115 L304 L305 L306 L307 | L115 L116 L117 L118 L304 | L146 L147 L148 L149 L151 L153 L154 L155 L156 L157 L158 L160 L213 L214 | L147 L149 L150 L151 L152 L153 L156 L157 L159 L215 picked at (7.6197, 33.677) makes body 1
extrude "Extrusion1" add sketch "Skizze1" along normal blind 2 separate body contours L0 L1 L2 L3 S0 L4 S1 L5 L6 L7 L8 L9 L10 L15 L24 L27 L29 L30 L31 A6 L32 L33 L40 L41 L42 L227 | L131 L133 L134 L135 L137 L139 L141 L144 L145 L161 L162 L166 L167 L169 L170 L171 L172 L176 L177 L178 L180 L218 | L131 L132 L133 L136 L137 L138 L139 L140 L141 L142 L143 L144 L162 L163 L164 L165 L166 L168 L169 L170 L172 L173 L174 L175 L176 L177 L179 L180 L219 | L43 L44 L45 L46 L252 | L45 L252 L253 L254 L255 | L47 L48 L49 L50 L248 | L50 L248 L249 L250 L251 | L51 L240 L241 L242 L243 | L51 L52 L53 L54 L240 | L55 L56 L57 L58 L236 | L58 L236 L237 L238 L239 | L59 L60 L61 L62 L232 | L62 L232 L233 L234 L235 | L63 L64 L65 L66 L256 | L66 L256 L257 L258 L259 | L67 L260 L261 L262 L263 | L67 L68 L69 L70 L260 | L71 L72 L73 L74 L264 | L72 L264 L265 L266 L267 | L75 L312 L313 L314 L315 | L75 L76 L77 L78 L312 | L79 L228 L229 L230 L231 | L79 L80 L81 L82 L228 | L119 L244 L245 L246 L247 | L119 L120 L121 L122 L244 | L123 L268 L269 L270 L271 | L123 L124 L125 L126 L268 | L127 L272 L273 L274 L275 | L127 L128 L129 L130 L272 | L184 L185 L186 L188 L189 L191 L223 | L181 L182 L183 L184 L186 L187 L188 L190 L191 L222 makes body 2
extrude "Extrusion12" cut sketch "Skizze1" along normal blind 2 from surface at 0.5 contours L111 L112 L114 L225 L308 | L111 L113 L114 L225 L308 | L111 L225 L308 L310 L311 | A0 | A1 | A2 | A3 | A4 | A5 | A9 | A11 | A12 | A13 | A15 L205 L208 | A15 L204 L205 L208 L210 | A15 L204 L210 | A16 | L43 L44 L45 L46 L252 | L45 L252 L253 L254 L255 | L47 L48 L49 L50 L248 | L50 L248 L249 L250 L251 | L51 L240 L241 L242 L243 | L51 L52 L53 L54 L240 | L55 L56 L57 L58 L236 | L58 L236 L237 L238 L239 | L59 L60 L61 L62 L232 | L62 L232 L233 L234 L235 | L63 L64 L65 L66 L256 | L66 L256 L257 L258 L259 | L67 L260 L261 L262 L263 | L67 L68 L69 L70 L260 | A17 | L71 L72 L73 L74 L264 | L72 L264 L265 L266 L267 | A18 | A19 | L75 L312 L313 L314 L315 | L75 L76 L77 L78 L312 | A20 | L79 L228 L229 L230 L231 | L79 L80 L81 L82 L228 | A21 | L83 L84 L85 L86 L276 | L86 L276 L277 L278 L279 | A22 | A23 | L87 L88 L89 L90 L280 | L90 L280 L281 L282 L283 | A24 | L91 L92 L93 L94 L284 | L94 L284 L285 L286 L287 | A25 | L95 L96 L97 L98 L288 | L98 L288 L289 L290 L291 | A26 | L99 L292 L293 L294 L295 | L99 L100 L101 L102 L292 | A27 | L103 L296 L297 L298 L299 | L103 L104 L105 L106 L296 | L107 L108 L109 L110 L300 | L110 L300 L301 L302 L303 | A28 | L115 L304 L305 L306 L307 | L115 L116 L117 L118 L304 | A29 | L119 L244 L245 L246 L247 | L119 L120 L121 L122 L244 | L123 L268 L269 L270 L271 | L123 L124 L125 L126 L268 | L127 L272 L273 L274 L275 | L127 L128 L129 L130 L272 bodies 1 2
extrude "Extrusion13" add sketch "Skizze1" along normal blind 10 contours L194 L195 L196 L198 L200 L201 L203 L205 L207 L208 | L192 L193 L194 L196 L197 L198 L199 L200 L202 L204 L209 L210 | L146 L147 L148 L149 L151 L153 L154 L155 L156 L157 L158 L160 L213 L214 | L147 L149 L150 L151 L152 L153 L156 L157 L159 L215 bodies 1
extrude "Extrusion14" add sketch "Skizze1" along normal blind 10 contours L131 L133 L134 L135 L137 L139 L141 L144 L145 L161 L162 L166 L167 L169 L170 L171 L172 L176 L177 L178 L180 L218 | L131 L132 L133 L136 L137 L138 L139 L140 L141 L142 L143 L144 L162 L163 L164 L165 L166 L168 L169 L170 L172 L173 L174 L175 L176 L177 L179 L180 L219 | L184 L185 L186 L188 L189 L191 L223 | L181 L182 L183 L184 L186 L187 L188 L190 L191 L222 bodies 2
mirror "Mirror1" about plane through (0, 0, 0) normal (1, 0, 0) of bodies 1 2 makes body 3 at (80.8893, 48.6463, 0) makes body 4 at (-77.9138, 59.3163, 0)
named bodies: "Rechts (1)", "Links (1)", "Rechts", "Links"
